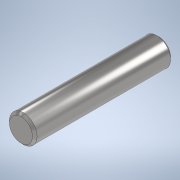
# Autodesk Inventor part: Штрифт
Saved by Autodesk Inventor 2021 (Build 250183000, 183)
## iProperties
Created: 2023-04-15
Part Number: Штрифт
Material: Сталь, углеродистая
Document SubType Name: Modeling
Designer: gdevc
Density: 7.85 g/cm^3
Appearance: С умеренной полировкой
Author: gdevc
Autodesk Inventor part; units mm, degrees
ref_plane "YZ Plane" through (0, 0, 0) normal (1, 0, 0) x (0, 1, 0)
ref_plane "XZ Plane" through (0, 0, 0) normal (0, 1, 0) x (-1, 0, 0)
ref_plane "XY Plane" through (0, 0, 0) normal (0, 0, 1) x (1, 0, 0)
sketch "Эскиз1" plane through (0, 0, 0) normal (0, 0, 1) x (1, 0, 0)
  circle A0 centre (0, 0) radius 3
  dimension "d0" = 6
  constraints: 1 centre point, 1 coincident
  measures "d0" diameter of A0
extrude "Выдавливание1" add sketch "Эскиз1" along normal blind 30
chamfer "Фаска1" distance 0.5 angle 45 1 edges at (-3, 0, 30)
chamfer "Фаска2" distance 0.5 angle 45 1 edges at (-3, 0, 0)
